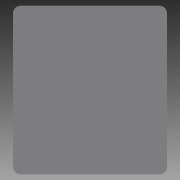
# Autodesk Inventor part: wall-end
Saved by Autodesk Inventor 2015 (Build 190159000, 159)
## iProperties
Created: 2014-07-16
Part Number: wall-end
Material: Generic
Document SubType Name: Modeling
Designer: pc
Density: 1 g/cm^3
Appearance: Default
Author: pc
Autodesk Inventor part; units mm, degrees
ref_plane "YZ Plane" through (0, 0, 0) normal (1, 0, 0) x (0, 1, 0)
ref_plane "XZ Plane" through (0, 0, 0) normal (0, 1, 0) x (-1, 0, 0)
ref_plane "XY Plane" through (0, 0, 0) normal (0, 0, 1) x (1, 0, 0)
sketch "Sketch1" plane through (0, 0, 0) normal (0, 1, 0) x (-1, 0, 0)
  line L0 (-21, 23) -> (21, 23)
  line L1 (21, 23) -> (21, -23)
  line L2 (21, -23) -> (-21, -23)
  line L3 (-21, -23) -> (-21, 23)
  line L4 (-21, 23) -> (21, -23) construction
  line L5 (21, 23) -> (-21, -23) construction
  point P0 (0, 0)
  dimension "d0" = 42
  dimension "d1" = 46
  constraints: 12 end point, 2 midpoint, 2 parallel, 1 horizontal, 1 perpendicular
  measures "d0" distance of L1.end L2.end
  measures "d1" distance of L0.end L1.end
extrude "wall3" add sketch "Sketch1" along normal blind 4
fillet "Fillet6" radius 2 1 edges at (-21, 2, -23)
fillet "Fillet7" radius 2 1 edges at (21, 2, -23)
fillet "Fillet8" radius 2 1 edges at (-21, 2, 23)
fillet "Fillet9" radius 2 1 edges at (21, 2, 23)
sketch "Sketch10" plane through (0, 4, 0) normal (0, 1, 0) x (1, 0, 0)
  line L0 (-20.8799, 11) -> (21, 11) construction
  line L1 (21, -21) -> (21, 21) projected
  line L2 (14.0018, 23) -> (14.0018, -23) construction
  line L3 (-19, -23) -> (19, -23) projected
  line L4 (19, 23) -> (-19, 23) projected
  line L5 (-21, 21) -> (18, 21)
  line L6 (18, 21) -> (18, 1)
  line L7 (18, 1) -> (-21, 1)
  line L8 (-21, 1) -> (-21, 21)
  line L9 (-21, 21) -> (18, 1) construction
  line L10 (18, 21) -> (-21, 1) construction
  line L11 (-21, 21) -> (-21, -21) projected
  point P0 (0, 0)
  point P1 (-1.5, 11)
  dimension "d98" = 34
  dimension "d99" = 20
  dimension "d100" = 3
  constraints: 16 end point, 4 point on line, 2 horizontal, 2 midpoint, 2 parallel, 1 collinear, 1 perpendicular, 1 vertical
  measures "d98" distance between parallel lines of L3 L0
  measures "d99" distance of L7.end L5.start
  measures "d100" distance between parallel lines of L1 L6
extrude "Extrusion8" cut sketch "Sketch10" against normal blind 2
equation "\"d0\" = wallw"
equation "\"d72\" = wall3_thick"
equation "\"d89\" = cornerrad"
equation "\"d90\" = cornerrad"
equation "\"d91\" = cornerrad"
equation "\"d92\" = cornerrad"
equation "\"d98\" = distancefrombottom"
equation "\"d99\" = wall3sloth"
equation "\"d100\" = -0.5 * wall3slotw + 0.5 * wallw"
equation "\"d101\" = wall3slotd"
equation "\"printer3dtolerance\" = 0.12"
equation "\"wallw\" = 42"
equation "\"wallh\" = 44"
equation "\"cornerrad\" = 2"
equation "\"baseextra\" = 2"
equation "\"wall1_thick\" = 8"
equation "\"wall2_thick\" = 6.4"
equation "\"wall3_thick\" = 4"
equation "\"wall1slot\" = 8.12"
equation "\"wall2slot\" = 6.52"
equation "\"wall3slot\" = 4.12"
equation "\"gap2\" = 28"
equation "\"baseh\" = 79.12"
equation "\"basew\" = 44"
equation "\"base_thick\" = 6"
equation "\"base_slots_depth\" = 4"
equation "\"servomounth\" = 4"
equation "\"servosmallcircledia\" = 5.92"
equation "\"servomountsquare\" = 6"
equation "\"servobigcircledia\" = 11.62"
equation "\"servo9gw\" = 22.8"
equation "\"distancefromleft\" = 26"
equation "\"servopolygonl\" = 5.92"
equation "\"servopolygonr\" = 6.12"
equation "\"distancefrombottom\" = 34"
equation "\"d49\" = distancefrombottom"
equation "\"adapterh\" = 16"
equation "\"adapterw\" = 32"
equation "\"wall3sloth\" = 20"
equation "\"wall3slotw\" = 36"
equation "\"wall3slotd\" = 2"
body "Solid2"
